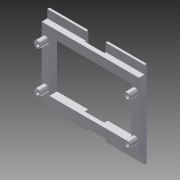
# Autodesk Inventor part: Heatsink al base
Saved by Autodesk Inventor 2015 (Build 190159000, 159)
## iProperties
Created: 2015-08-21
Part Number: Heatsink al base
Material: Aluminum 6061
Document SubType Name: Modeling
Designer: Kyle
Density: 2.7 g/cm^3
Appearance: Aluminum - Flat
Author: Kyle
Autodesk Inventor part; units mm, degrees
ref_plane "YZ Plane" through (0, 0, 0) normal (1, 0, 0) x (0, 1, 0)
ref_plane "XZ Plane" through (0, 0, 0) normal (0, 1, 0) x (-1, 0, 0)
ref_plane "XY Plane" through (0, 0, 0) normal (0, 0, 1) x (1, 0, 0)
sketch "Sketch1" plane through (0, 0, 0) normal (0, 0, 1) x (1, 0, 0)
  line L0 (0, 0) -> (88.9, 0)
  line L1 (88.9, 0) -> (88.9, -63.5)
  line L2 (88.9, -63.5) -> (0, -63.5)
  line L3 (0, -63.5) -> (0, 0)
  line L4 (6.985, -8.255) -> (81.915, -8.255)
  line L5 (81.915, -8.255) -> (81.915, -55.245)
  line L6 (81.915, -55.245) -> (6.985, -55.245)
  line L7 (6.985, -55.245) -> (6.985, -8.255)
  dimension "d0" = 88.9
  dimension "d1" = 63.5
  dimension "d2" = 8.255
  dimension "d3" = 8.255
  dimension "d4" = 6.985
  dimension "d5" = 6.985
  constraints: 16 end point, 4 parallel, 2 horizontal, 2 perpendicular
  measures "d0" distance of L0.start L0.end
  measures "d1" distance of L2.end L0.start
  measures "d2" distance between parallel lines of L0 L4
  measures "d3" distance between parallel lines of L2 L6
  measures "d4" distance between parallel lines of L3 L7
  measures "d5" distance between parallel lines of L1 L5
extrude "Extrusion1" add sketch "Sketch1" along normal blind 5.08
sketch "Sketch2" plane through (0, 0, 5.08) normal (0, 0, 1) x (1, 0, 0)
  circle A0 centre (3.4925, -12.7) radius 3.175
  circle A1 centre (3.4925, -50.8) radius 3.175
  circle A2 centre (85.4075, -50.8) radius 3.175
  circle A3 centre (85.4075, -12.7) radius 3.175
  line L0 (88.9, 0) -> (0, 0) projected
  line L1 (0, -63.5) -> (88.9, -63.5) projected
  line L2 (0, 0) -> (0, -63.5) projected
  line L3 (81.915, -8.255) -> (81.915, -55.245) projected
  circle A4 centre (85.4075, -50.8) radius 1.905
  circle A5 centre (85.4075, -12.7) radius 1.905
  circle A6 centre (3.4925, -50.8) radius 1.905
  circle A7 centre (3.4925, -12.7) radius 1.905
  dimension "d8" = 6.35
  dimension "d9" = 6.35
  dimension "d10" = 6.35
  dimension "d11" = 6.35
  dimension "d12" = 12.7
  dimension "d13" = 12.7
  dimension "d14" = 12.7
  dimension "d15" = 12.7
  dimension "d16" = 3.4925
  dimension "d17" = 3.4925
  dimension "d18" = 3.81
  constraints: 8 centre point, 4 coincident
  measures "d8" diameter of A0
  measures "d9" diameter of A1
  measures "d10" diameter of A2
  measures "d11" diameter of A3
  measures "d12" distance from line of A3.centre L0
  measures "d13" distance from line of L1 A2.centre
  measures "d14" distance from line of L0 A0.centre
  measures "d15" distance from line of A1.centre L1
  measures "d16" distance from line of L2 A0.centre
  measures "d17" distance from line of L3 A3.centre
  measures "d18" diameter of A4
extrude "Extrusion2" add sketch "Sketch2" along normal blind 7.62
sketch "Sketch3" plane through (0, 0, 0) normal (0, 0, -1) x (-1, 0, 0)
  line L0 (0, 7.62) -> (0, -71.12)
  line L1 (-88.9, -71.12) -> (-88.9, 7.62)
  line L2 (0, 0) -> (-88.9, 0) projected
  line L3 (-88.9, -63.5) -> (0, -63.5) projected
  line L4 (-88.9, 0) -> (-88.9, -63.5) projected
  line L5 (0, -63.5) -> (0, 0) projected
  line L6 (-35.56, 0) -> (-35.56, 7.62)
  line L7 (-53.34, 7.62) -> (-53.34, 0)
  line L8 (0, -63.5) -> (-88.9, -63.5) projected
  line L9 (-53.34, -63.5) -> (-53.34, -71.12)
  line L10 (-35.56, -63.5) -> (-35.56, -71.12)
  line L11 (-88.9, 7.62) -> (-53.34, 7.62)
  line L12 (-35.56, 7.62) -> (0, 7.62)
  line L13 (0, -71.12) -> (-35.56, -71.12)
  line L14 (-53.34, -71.12) -> (-88.9, -71.12)
  point P0 (-88.9, -31.75)
  point P1 (0, -31.75)
  dimension "d23" = 35.56
  dimension "d24" = 35.56
  constraints: 20 end point, 6 perpendicular, 5 parallel, 4 midpoint, 4 point on line, 2 horizontal, 2 vertical
  measures "d23" distance between parallel lines of L0 L6
  measures "d24" distance between parallel lines of L1 L7
extrude "Extrusion3" add sketch "Sketch3" along normal blind 1.905
sketch "Sketch4" plane through (0, 0, 0) normal (0, 0, 1) x (1, 0, 0)
  line L0 (6.985, -8.255) -> (81.915, -8.255)
  line L1 (81.915, -8.255) -> (81.915, -55.245)
  line L2 (81.915, -55.245) -> (6.985, -55.245)
  line L3 (6.985, -55.245) -> (6.985, -8.255)
  point P0 (0, 0)
  constraints: 8 end point, 2 parallel, 1 horizontal, 1 perpendicular
extrude "Extrusion4" cut sketch "Sketch4" against normal blind 1.905
sketch "Sketch5" plane through (0, 0, -1.905) normal (0, 0, -1) x (-1, 0, 0)
  line L0 (0, -63.5) -> (-88.9, -63.5) projected
  line L1 (-53.34, 0) -> (-35.56, 0)
  line L2 (-35.56, 0) -> (-35.56, -63.5)
  line L3 (-35.56, -63.5) -> (-53.34, -63.5)
  line L4 (-53.34, -63.5) -> (-53.34, 0)
  point P0 (0, 0)
  dimension "d29" = 17.78
  constraints: 8 end point, 2 parallel, 1 horizontal, 1 perpendicular, 1 point on line
  measures "d29" distance between parallel lines of L2 L4
extrude "Extrusion5" cut sketch "Sketch5" against normal blind 3.175
sketch "Sketch6" plane through (85.4075, -12.7, 12.7) normal (0, 0, 1) x (1, 0, 0)
  circle A0 centre (0, 0) radius 1.905
  circle A1 centre (-81.915, 0) radius 1.905 projected
  circle A2 centre (-81.915, 0) radius 1.905
  circle A3 centre (0, -38.1) radius 1.905 projected
  circle A4 centre (0, -38.1) radius 1.905
  circle A5 centre (-81.915, -38.1) radius 1.905 projected
  circle A6 centre (-81.915, -38.1) radius 1.905
  point P0 (-85.4075, 12.7)
  constraints: 4 centre point, 3 coincident
extrude "Extrusion6" cut sketch "Sketch6" against normal blind 25.4
body "Solid1"
